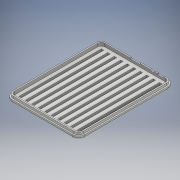
# Autodesk Inventor part: CaseGroboyBackSlatHoriz
Saved by Autodesk Inventor 2017 SP1 (Build 210196100, 196)
## iProperties
Created: 2017-08-23
Part Number: CaseGroboyBackSlatHoriz
Material: Generic
Document SubType Name: Modeling
Designer: Groguard
Density: 1 g/cm^3
Appearance: Default
Author: Groguard
Autodesk Inventor part; units mm, degrees
ref_plane "YZ Plane" through (0, 0, 0) normal (1, 0, 0) x (0, 1, 0)
ref_plane "XZ Plane" through (0, 0, 0) normal (0, 1, 0) x (-1, 0, 0)
ref_plane "XY Plane" through (0, 0, 0) normal (0, 0, 1) x (1, 0, 0)
sketch "Sketch6" plane through (0, 0, 0) normal (0, 0, 1) x (1, 0, 0)
  arc A0 (83, 106.5858) -> (78.5858, 111) centre (78.5858, 106.5858) ccw
  line L0 (83, 106.5858) -> (83, 3.4142)
  arc A1 (78.5858, -1) -> (83, 3.4142) centre (78.5858, 3.4142) ccw
  line L1 (78.5858, -1) -> (3.4142, -1)
  arc A2 (-1, 3.4142) -> (3.4142, -1) centre (3.4142, 3.4142) ccw
  line L2 (-1, 3.4142) -> (-1, 106.5858)
  arc A3 (3.4142, 111) -> (-1, 106.5858) centre (3.4142, 106.5858) ccw
  line L3 (3.4142, 111) -> (78.5858, 111)
  arc A4 (86, 106.5858) -> (78.5858, 114) centre (78.5858, 106.5858) ccw
  line L4 (86, 106.5858) -> (86, 3.4142)
  arc A5 (78.5858, -4) -> (86, 3.4142) centre (78.5858, 3.4142) ccw
  line L5 (78.5858, -4) -> (3.4142, -4)
  arc A6 (-4, 3.4142) -> (3.4142, -4) centre (3.4142, 3.4142) ccw
  line L6 (-4, 3.4142) -> (-4, 106.5858)
  arc A7 (3.4142, 114) -> (-4, 106.5858) centre (3.4142, 106.5858) ccw
  line L7 (3.4142, 114) -> (78.5858, 114)
  constraints: 16 end point, 16 point on circle, 8 centre point
extrude "Extrusion4" add sketch "Sketch6" along normal blind 3 contours L0 A1 L1 A2 L2 A3 L3 A0 | L4 A5 L5 A6 L6 A7 L7 A4
sketch "Sketch7" plane through (0, 0, 3) normal (0, 0, 1) x (1, 0, 0)
  line L0 (83, 106.5858) -> (83, 3.4142)
  line L1 (-1, 3.4142) -> (-1, 106.5858)
  arc A0 (78.5858, -1) -> (83, 3.4142) centre (78.5858, 3.4142) ccw
  arc A1 (-1, 3.4142) -> (3.4142, -1) centre (3.4142, 3.4142) ccw
  line L2 (78.5858, -1) -> (3.4142, -1)
  line L3 (3.4142, 111) -> (78.5858, 111)
  arc A2 (3.4142, 111) -> (-1, 106.5858) centre (3.4142, 106.5858) ccw
  arc A3 (83, 106.5858) -> (78.5858, 111) centre (78.5858, 106.5858) ccw
  line L4 (-4, 106.5858) -> (-4, 3.4142)
  arc A4 (-4, 3.4142) -> (3.4142, -4) centre (3.4142, 3.4142) ccw
  line L5 (3.4142, -4) -> (78.5858, -4)
  arc A5 (78.5858, -4) -> (86, 3.4142) centre (78.5858, 3.4142) ccw
  line L6 (86, 3.4142) -> (86, 106.5858)
  arc A6 (86, 106.5858) -> (78.5858, 114) centre (78.5858, 106.5858) ccw
  line L7 (78.5858, 114) -> (3.4142, 114)
  arc A7 (3.4142, 114) -> (-4, 106.5858) centre (3.4142, 106.5858) ccw
  point P0 (0, 0)
  dimension "d17" = 3
  constraints: 16 end point, 16 point on circle, 8 centre point, 7 other
  measures "d17" radial gap between concentric circles of A2 A7
extrude "Extrusion5" add sketch "Sketch7" along normal blind 4
sketch "Sketch8" plane through (0, 0, 7) normal (0, 0, 1) x (1, 0, 0)
  arc A0 (3.4142, 111) -> (-1, 106.5858) centre (3.4142, 106.5858) ccw
  line L0 (3.4142, 111) -> (78.5858, 111)
  arc A1 (83, 106.5858) -> (78.5858, 111) centre (78.5858, 106.5858) ccw
  line L1 (-1, 3.4142) -> (-1, 106.5858)
  line L2 (83, 106.5858) -> (83, 3.4142)
  arc A2 (-1, 3.4142) -> (3.4142, -1) centre (3.4142, 3.4142) ccw
  line L3 (78.5858, -1) -> (3.4142, -1)
  arc A3 (78.5858, -1) -> (83, 3.4142) centre (78.5858, 3.4142) ccw
  line L4 (-4, 106.5858) -> (-4, 3.4142)
  arc A4 (-4, 3.4142) -> (3.4142, -4) centre (3.4142, 3.4142) ccw
  line L5 (3.4142, -4) -> (78.5858, -4)
  arc A5 (78.5858, -4) -> (86, 3.4142) centre (78.5858, 3.4142) ccw
  line L6 (86, 3.4142) -> (86, 106.5858)
  arc A6 (86, 106.5858) -> (78.5858, 114) centre (78.5858, 106.5858) ccw
  line L7 (78.5858, 114) -> (3.4142, 114)
  arc A7 (3.4142, 114) -> (-4, 106.5858) centre (3.4142, 106.5858) ccw
  line L8 (-2.5, 106.5858) -> (-2.5, 3.4142)
  arc A8 (-2.5, 3.4142) -> (3.4142, -2.5) centre (3.4142, 3.4142) ccw
  line L9 (3.4142, -2.5) -> (78.5858, -2.5)
  arc A9 (78.5858, -2.5) -> (84.5, 3.4142) centre (78.5858, 3.4142) ccw
  line L10 (84.5, 3.4142) -> (84.5, 106.5858)
  arc A10 (84.5, 106.5858) -> (78.5858, 112.5) centre (78.5858, 106.5858) ccw
  line L11 (78.5858, 112.5) -> (3.4142, 112.5)
  arc A11 (3.4142, 112.5) -> (-2.5, 106.5858) centre (3.4142, 106.5858) ccw
  point P0 (0, 0)
  point P1 (0, 0)
  dimension "d20" = 3
  dimension "d21" = 1.5
  constraints: 24 end point, 24 point on circle, 12 centre point, 14 other
  measures "d20" radial gap between concentric circles of A0 A7
  measures "d21" radial gap between concentric circles of A7 A11
extrude "Extrusion6" cut sketch "Sketch8" against normal blind 3 contours A7 L7 A6 L6 A5 L5 A4 L4
fillet "Fillet2" radius 2 8 edges at (-1.8284, 111.8284, 0) (-4, 55, 0) (-1.8284, -1.8284, 0) (41, -4, 0) (83.8284, -1.8284, 0) (86, 55, 0) (83.8284, 111.8284, 0) (41, 114, 0)
sketch "Sketch9" plane through (3.4142, 111, 3) normal (0, -1, 0) x (1, 0, 0)
  line L0 (73.1716, 4) -> (65.1716, 4)
  line L1 (65.1716, 4) -> (73.1716, 4)
  line L2 (73.1716, 4) -> (73.1716, 3)
  line L3 (73.1716, 3) -> (65.1716, 3)
  line L4 (65.1716, 3) -> (65.1716, 4)
  circle A0 centre (59.1716, 6) radius 3.25
  line L5 (37.5858, 4) -> (37.5858, 3)
  line L6 (31.5858, 5) -> (43.5858, 5)
  line L7 (43.5858, 5) -> (43.5858, 3)
  line L8 (43.5858, 3) -> (31.5858, 3)
  line L9 (31.5858, 3) -> (31.5858, 5)
  line L10 (31.5858, 5) -> (43.5858, 3) construction
  line L11 (43.5858, 5) -> (31.5858, 3) construction
  dimension "d37" = 1
  dimension "d38" = 12
  constraints: 24 end point, 4 parallel, 2 horizontal, 2 midpoint, 2 perpendicular, 1 centre point, 1 vertical
  measures "d37" distance of L5.start L5.end
  measures "d38" distance of L7.end L8.end
extrude "Extrusion7" cut sketch "Sketch9" against normal blind 3
sketch "Sketch10" plane through (0, 0, 3) normal (0, 0, 1) x (1, 0, 0)
  line L0 (3.4142, 106.5858) -> (6.4142, 106.5858)
  line L1 (6.4142, 106.5858) -> (6.4142, 4.4379)
  line L2 (6.4142, 4.4379) -> (3.4142, 4.4379)
  line L3 (3.4142, 4.4379) -> (3.4142, 106.5858)
  line L4 (83, 3.4142) -> (83, 106.5858) projected
  line L5 (83, 55) -> (78.586, 55)
  line L6 (83, 55) -> (87.414, 55) construction
  line L7 (11.4342, 106.5858) -> (14.4342, 106.5858)
  line L8 (14.4342, 106.5858) -> (14.4342, 4.4379)
  line L9 (11.4342, 4.4379) -> (11.4342, 106.5858)
  line L10 (14.4342, 4.4379) -> (11.4342, 4.4379)
  line L11 (19.4542, 106.5858) -> (22.4542, 106.5858)
  line L12 (22.4542, 106.5858) -> (22.4542, 4.4379)
  line L13 (19.4542, 4.4379) -> (19.4542, 106.5858)
  line L14 (22.4542, 4.4379) -> (19.4542, 4.4379)
  line L15 (27.4742, 106.5858) -> (30.4742, 106.5858)
  line L16 (30.4742, 106.5858) -> (30.4742, 4.4379)
  line L17 (27.4742, 4.4379) -> (27.4742, 106.5858)
  line L18 (30.4742, 4.4379) -> (27.4742, 4.4379)
  line L19 (35.4942, 106.5858) -> (38.4942, 106.5858)
  line L20 (38.4942, 106.5858) -> (38.4942, 4.4379)
  line L21 (35.4942, 4.4379) -> (35.4942, 106.5858)
  line L22 (38.4942, 4.4379) -> (35.4942, 4.4379)
  line L23 (43.5142, 106.5858) -> (46.5142, 106.5858)
  line L24 (46.5142, 106.5858) -> (46.5142, 4.4379)
  line L25 (43.5142, 4.4379) -> (43.5142, 106.5858)
  line L26 (46.5142, 4.4379) -> (43.5142, 4.4379)
  line L27 (51.5342, 106.5858) -> (54.5342, 106.5858)
  line L28 (54.5342, 106.5858) -> (54.5342, 4.4379)
  line L29 (51.5342, 4.4379) -> (51.5342, 106.5858)
  line L30 (54.5342, 4.4379) -> (51.5342, 4.4379)
  line L31 (59.5542, 106.5858) -> (62.5542, 106.5858)
  line L32 (62.5542, 106.5858) -> (62.5542, 4.4379)
  line L33 (59.5542, 4.4379) -> (59.5542, 106.5858)
  line L34 (62.5542, 4.4379) -> (59.5542, 4.4379)
  line L35 (67.5742, 106.5858) -> (70.5742, 106.5858)
  line L36 (70.5742, 106.5858) -> (70.5742, 4.4379)
  line L37 (67.5742, 4.4379) -> (67.5742, 106.5858)
  line L38 (70.5742, 4.4379) -> (67.5742, 4.4379)
  line L39 (75.5942, 106.5858) -> (78.5942, 106.5858)
  line L40 (78.5942, 106.5858) -> (78.5942, 4.4379)
  line L41 (75.5942, 4.4379) -> (75.5942, 106.5858)
  line L42 (78.5942, 4.4379) -> (75.5942, 4.4379)
  dimension "d41" = 3
  dimension "d42" = 4.414
  dimension "d43" = 180
  dimension "d49" = 8.02
  constraints: 84 end point, 4 horizontal, 2 collinear, 2 parallel, 1 midpoint, 1 perpendicular, 71 other
  measures "d41" distance of L1.end L2.end
  measures "d42" distance of L5.start L5.end
  measures "d43" angle of L5 L6
  measures "d49" distance of L0.start L7.start
extrude "Extrusion8" cut sketch "Sketch10" against normal blind 3
body "Solid2"
